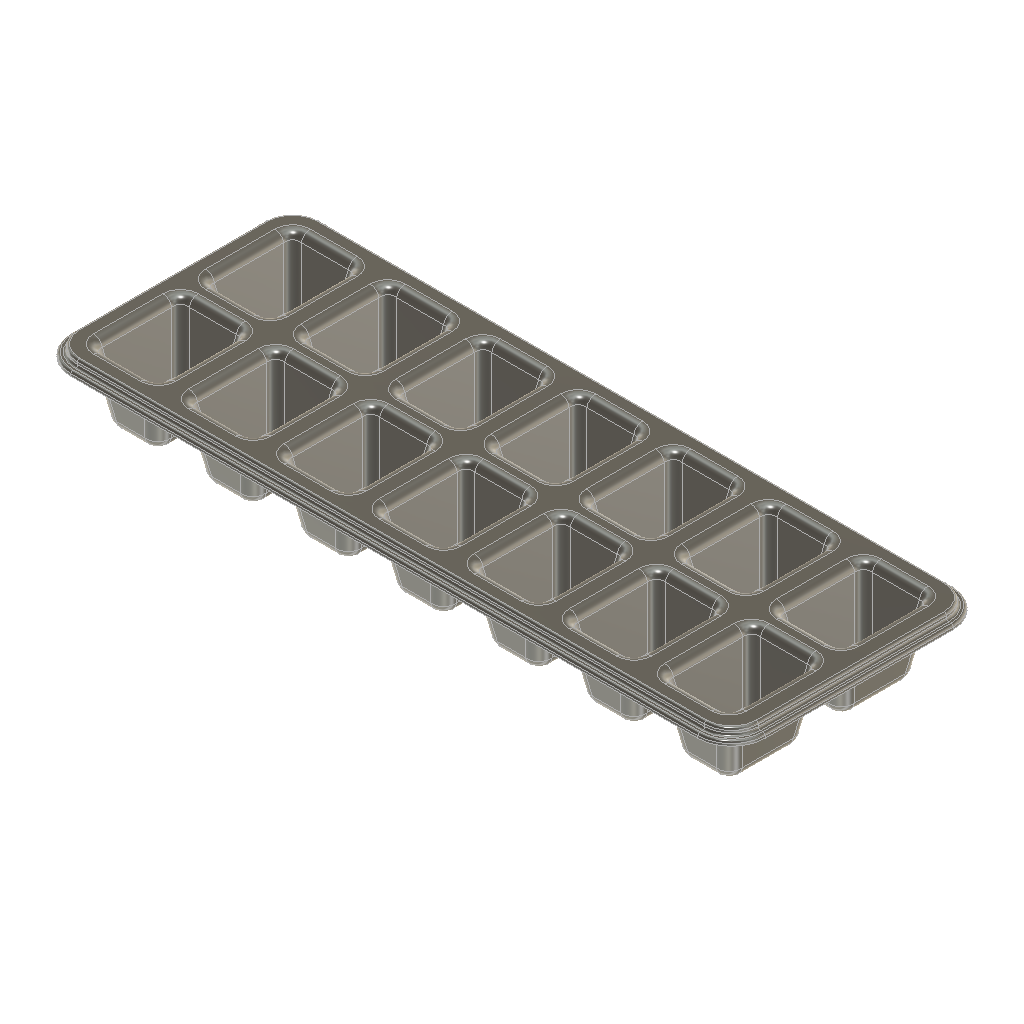
Ice Cube Tray (Autodesk Fusion 360 design; units mm, degrees)
part number: 2026-09-26-20-22-52-773
Autodesk Fusion 360 part; units mm, degrees
sketch "Sketch1" plane through (0, 0, 0) normal (0, 0, 1) x (1, 0, 0)
  line L0 (150, 52) -> (-150, 52)
  line L1 (-150, 52) -> (-150, -52)
  line L2 (-150, -52) -> (150, -52)
  line L3 (150, -52) -> (150, 52)
  line L4 (150, 52) -> (-150, -52) construction
  line L5 (-150, 52) -> (150, -52) construction
  dimension "d1" = 300
  dimension "d2" = 104
  constraint horizontal L0
  constraint perpendicular L0 L1
  constraint parallel L0 L2
  constraint parallel L1 L3
  constraint coincident L4 origin
  constraint coincident L5 origin
  measures "d1" distance of L1.end L2.end
  measures "d2" distance of L0.end L1.end
extrude "Extrude1" add sketch "Sketch1" along normal blind 50
sketch "Sketch2" plane through (0, 0, 50) normal (0, 0, 1) x (-1, 0, 0)
  line L0 (-150, 52) -> (-150, -52)
  line L1 (-150, -52) -> (150, -52)
  line L2 (150, -52) -> (150, 52)
  line L3 (150, 52) -> (-150, 52)
  line L4 (143, -45) -> (113, -45)
  line L5 (113, -45) -> (113, -5)
  line L6 (113, -5) -> (143, -5)
  line L7 (143, -5) -> (143, -45)
  dimension "d5" = 30
  dimension "d6" = 40
  dimension "d7" = 7
  dimension "d8" = 7
  constraint horizontal L4
  constraint vertical L5
  constraint horizontal L6
  constraint vertical L7
  measures "d5" distance of L4.start L4.end
  measures "d6" distance of L4.start L6.end
  measures "d7" distance of L1 L4
  measures "d8" distance of L2 L7
extrude "Extrude2" cut sketch "Sketch2" against normal blind 30 draft -10 contours L4 L5 L6 L7
fillet "Fillet1" radius 4 5 faces at (-131.2367, 43.2367, 40) (-141.2367, 20.0966, 40) (-124.7633, 20.0966, 20) (-114.7633, 29.9034, 40) (-124.7633, 6.7633, 40)
pattern_linear "R-Pattern1" count 7 spacing 42.5 along (1, 0, 0) count 2 spacing 50 along (0, -1, 0) of "Extrude2", "Fillet1"
shell "Shell2" thickness 2 removed faces 5 at (-50, -52, 16.6667) at (-150, 17.3333, 16.6667) at (50, 52, 16.6667) at (150, -17.3333, 16.6667) at (-50, -17.3333, 0)
fillet "Fillet2" radius 10 4 edges at (150, -52, 49) (150, 52, 49) (-150, 52, 49) (-150, -52, 49)
sketch "Sketch3" plane through (0, 0, 0) normal (0, 1, 0) x (1, 0, 0)
  line L0 (-150, -50) -> (-150, -45)
  line L1 (-150, -45) -> (-155, -45)
  line L2 (-155, -45) -> (-155, -47)
  line L3 (-155, -47) -> (-152, -47)
  line L4 (-152, -47) -> (-152, -50)
  line L5 (-152, -50) -> (-150, -50)
  point P0 (-150, -50)
  dimension "d21" = 2
  dimension "d22" = 3
  dimension "d23" = 5
  dimension "d24" = 2
  constraint vertical L0
  constraint perpendicular L0 L1
  constraint perpendicular L0 L3
  constraint perpendicular L1 L4
  constraint coincident P0 L0.start
  measures "d21" distance of P0 L4.end
  measures "d22" distance of L3.end L4.end
  measures "d23" distance of L0.end L1.end
  measures "d24" distance of L1.end L2.end
sweep "Sweep1" add profiles "Sketch3" along 8 edges at (147.0711, -49.0711, 50) (150, 0, 50) (147.0711, 49.0711, 50) (0, 52, 50) (-147.0711, 49.0711, 50) (-150, 0, 50) (-147.0711, -49.0711, 50) (0, -52, 50) section 1
fillet "Fillet3" radius 1 24 edges at (148.4853, -50.4853, 50) (152, 0, 50) (148.4853, 50.4853, 50) (0, 54, 50) (-148.4853, 50.4853, 50) (-152, 0, 50) (-148.4853, -50.4853, 50) (0, -54, 50) (148.4853, -50.4853, 47) (152, 0, 47) (148.4853, 50.4853, 47) (0, 54, 47) (-148.4853, 50.4853, 47) (-152, 0, 47) (-148.4853, -50.4853, 47) (0, -54, 47) (150.6066, -52.6066, 47) (155, 0, 47) (150.6066, 52.6066, 47) (0, 57, 47) (-150.6066, 52.6066, 47) (-155, 0, 47) (-150.6066, -52.6066, 47) (0, -57, 47)
equation "d8 = d7"
